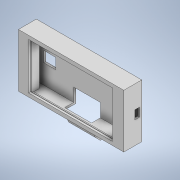
# Autodesk Inventor part: left
Saved by Autodesk Inventor 2020 (Build 240168000, 168)
## iProperties
Created: 2021-08-13
Part Number: left
Material: Generic
Document SubType Name: Modeling
Designer: khonsu
Density: 1 g/cm^3
Appearance: Default
Author: khonsu
Autodesk Inventor part; units mm, degrees
ref_plane "YZ Plane" through (0, 0, 0) normal (1, 0, 0) x (0, 1, 0)
ref_plane "XZ Plane" through (0, 0, 0) normal (0, 1, 0) x (-1, 0, 0)
ref_plane "XY Plane" through (0, 0, 0) normal (0, 0, 1) x (1, 0, 0)
sketch "Sketch1" plane through (0, 0, 0) normal (0, 0, 1) x (1, 0, 0)
  line L0 (0, 0) -> (74, 0)
  line L1 (74, 0) -> (74, -7.6)
  line L2 (74, -7.6) -> (0, -7.6)
  line L3 (0, -7.6) -> (0, 0)
  line L4 (0.9, 13.2) -> (73.1, 13.2)
  line L5 (73.1, 13.2) -> (73.1, 12)
  line L6 (73.1, 12) -> (0.9, 12)
  line L7 (0.9, 12) -> (0.9, 13.2)
  line L8 (-3, 16.2) -> (77, 16.2)
  line L9 (77, 16.2) -> (77, -10.6)
  line L10 (77, -10.6) -> (-3, -10.6)
  line L11 (-3, -10.6) -> (-3, 16.2)
  dimension "d0" = 74
  dimension "d1" = 7.6
  dimension "d2" = 1.2
  dimension "d3" = 12
  dimension "d4" = 72.2
  dimension "d5" = 0.9
  dimension "d6" = 3
  dimension "d7" = 3
  dimension "d8" = 3
  dimension "d9" = 3
  constraints: 24 end point, 6 parallel, 3 horizontal, 3 perpendicular
  measures "d0" distance of L0.start L0.end
  measures "d1" distance of L0.end L1.end
  measures "d2" distance of L4.end L5.end
  measures "d3" distance between parallel lines of L0 L6
  measures "d4" distance of L4.start L4.end
  measures "d5" distance between parallel lines of L3 L7
  measures "d6" distance between parallel lines of L8 L4
  measures "d7" distance between parallel lines of L2 L10
  measures "d8" distance between parallel lines of L3 L11
  measures "d9" distance between parallel lines of L9 L1
extrude "Extrusion1" add sketch "Sketch1" along normal blind 151.5
sketch "Sketch2" plane through (-3, 16.2, 0) normal (0, 1, 0) x (1, 0, 0)
  line L0 (77, -12.1) -> (3, -12.1)
  line L1 (3, -12.1) -> (3, -137.5)
  line L2 (3, -137.5) -> (77, -137.5)
  line L3 (77, -137.5) -> (77, -12.1)
  line L4 (80, 0) -> (80, -151.5) projected
  line L5 (0, 0) -> (0, -151.5) projected
  line L6 (80, 0) -> (0, 0) projected
  line L7 (80, -151.5) -> (0, -151.5) projected
  point P0 (3, 0)
  dimension "d12" = 3
  dimension "d14" = 12.1
  dimension "d15" = 14
  dimension "d23" = 3
  constraints: 8 end point, 2 parallel, 1 horizontal, 1 perpendicular
  measures "d12" distance between parallel lines of L4 L3
  measures "d14" distance between parallel lines of L6 L0
  measures "d15" distance between parallel lines of L7 L2
  measures "d23" distance between parallel lines of L5 L1
extrude "Extrusion2" cut sketch "Sketch2" against normal up to surface (23.8 mm away) contours L3 L2 L1 L0
sketch "Sketch3" plane through (-3, 16.2, 0) normal (0, 1, 0) x (1, 0, 0)
  line L0 (80, 0) -> (80, -151.5) projected
  line L1 (0, 0) -> (0, -151.5) projected
  line L2 (80, -0.75) -> (0, -0.75)
  line L3 (0, -0.75) -> (0, -150.75)
  line L4 (0, -150.75) -> (80, -150.75)
  line L5 (80, -150.75) -> (80, -0.75)
  line L6 (80, -151.5) -> (0, -151.5) projected
  line L7 (80, 0) -> (0, 0) projected
  line L8 (80, 0) -> (0, 0)
  line L9 (0, 0) -> (0, -151.5)
  line L10 (0, -151.5) -> (80, -151.5)
  line L11 (80, -151.5) -> (80, 0)
  point P0 (3, 0)
  point P1 (0, -0.75)
  dimension "d18" = 150
  dimension "d19" = 151.5
  dimension "d20" = 0.75
  constraints: 16 end point, 4 parallel, 2 horizontal, 2 perpendicular, 2 point on line
  measures "d18" distance between parallel lines of L4 L2
  measures "d19" distance of L0.start L0.end
  measures "d20" distance between parallel lines of L6 L4
extrude "Extrusion3" add sketch "Sketch3" against normal up to surface (4.2 mm away) contours L0 L2 L1 L7 | L0 L6 L1 L4
sketch "Sketch4" plane through (0, 0, 0) normal (0, 0, -1) x (-1, 0, 0)
  line L0 (-77, -10.6) -> (-77, 16.2) projected
  line L1 (3, 16.2) -> (3, -10.6) projected
  line L2 (-77, -10.6) -> (3, -10.6)
  line L3 (3, -10.6) -> (3, 16.2)
  line L4 (3, 16.2) -> (-77, 16.2)
  line L5 (-77, 16.2) -> (-77, -10.6)
  point P0 (0, 0)
  constraints: 8 end point, 2 parallel, 1 horizontal, 1 perpendicular
extrude "Extrusion4" add sketch "Sketch4" along normal blind 3
sketch "Sketch5" plane through (0, 0, 151.5) normal (0, 0, 1) x (1, 0, 0)
  line L0 (-3, 16.2) -> (77, 16.2) projected
  line L1 (77, -10.6) -> (-3, -10.6) projected
  line L2 (77, 16.2) -> (-3, 16.2)
  line L3 (-3, 16.2) -> (-3, -10.6)
  line L4 (-3, -10.6) -> (77, -10.6)
  line L5 (77, -10.6) -> (77, 16.2)
  line L6 (43.5, -0.4) -> (30.5, -0.4)
  line L7 (30.5, -0.4) -> (30.5, -7.2)
  line L8 (30.5, -7.2) -> (43.5, -7.2)
  line L9 (43.5, -7.2) -> (43.5, -0.4)
  line L10 (74, -7.6) -> (0, -7.6) projected
  line L11 (74, 0) -> (74, -7.6) projected
  point P0 (0, 0)
  dimension "d26" = 6.8
  dimension "d27" = 13
  dimension "d28" = 0.4
  dimension "d29" = 30.5
  constraints: 16 end point, 4 parallel, 2 horizontal, 2 perpendicular
  measures "d26" distance of L8.end L6.start
  measures "d27" distance of L7.end L8.end
  measures "d28" distance between parallel lines of L10 L8
  measures "d29" distance between parallel lines of L11 L9
extrude "Extrusion5" add sketch "Sketch5" along normal blind 3
sketch "Sketch6" plane through (-3, -10.6, -3) normal (0, -1, 0) x (1, 0, 0)
  line L0 (48, 14.3) -> (32, 14.3)
  line L1 (32, 14.3) -> (32, 32)
  line L2 (32, 32) -> (48, 32)
  line L3 (48, 32) -> (48, 14.3)
  line L4 (77, 3) -> (3, 3) projected
  line L5 (80, 157.5) -> (80, 0) projected
  dimension "d32" = 11.3
  dimension "d33" = 16
  dimension "d34" = 17.7
  dimension "d35" = 32
  constraints: 8 end point, 2 parallel, 1 horizontal, 1 perpendicular
  measures "d32" distance between parallel lines of L4 L0
  measures "d33" distance of L0.start L0.end
  measures "d34" distance of L2.end L0.start
  measures "d35" distance between parallel lines of L5 L3
extrude "Extrusion6" cut sketch "Sketch6" against normal up to surface (3 mm away)
sketch "Sketch7" plane through (-3, 16.2, -3) normal (0, 1, 0) x (1, 0, 0)
  line L0 (3, -15.1) -> (77, -15.1) projected
  line L1 (77, -140.5) -> (3, -140.5) projected
  line L2 (74.6, -15.1) -> (5.4, -15.1)
  line L3 (5.4, -15.1) -> (5.4, -140.5)
  line L4 (5.4, -140.5) -> (74.6, -140.5)
  line L5 (74.6, -140.5) -> (74.6, -15.1)
  line L6 (77, -15.1) -> (77, -140.5) projected
  line L7 (3, -140.5) -> (3, -15.1) projected
  line L8 (77, -3) -> (77, -15.1) projected
  line L9 (77, -15.1) -> (3, -15.1)
  line L10 (3, -15.1) -> (3, -140.5)
  line L11 (3, -140.5) -> (77, -140.5)
  line L12 (77, -140.5) -> (77, -15.1)
  point P0 (3, -3)
  point P1 (5.4, -15.1)
  dimension "d38" = 2.4
  dimension "d39" = 2.4
  constraints: 16 end point, 4 parallel, 2 horizontal, 2 perpendicular, 2 point on line
  measures "d38" distance between parallel lines of L6 L5
  measures "d39" distance between parallel lines of L7 L3
extrude "Extrusion7" add sketch "Sketch7" against normal up to surface (3 mm away) contours L0 L3 L1 L7 | L0 L6 L1 L5
sketch "Sketch8" plane through (0, 0, -3) normal (0, 0, -1) x (-1, 0, 0)
  line L0 (-74, -7.6) -> (0, -7.6) projected
  line L1 (-18.5, -7.6) -> (-28.5, -7.6)
  line L2 (-31, -5.1) -> (-31, -5.1)
  line L3 (-28.5, -2.6) -> (-18.5, -2.6)
  line L4 (-16, -5.1) -> (-16, -5.1)
  line L5 (0, -7.6) -> (0, 0) projected
  line L6 (0, 0) -> (-74, 0) projected
  arc A0 (-31, -5.1) -> (-28.5, -7.6) centre (-28.5, -5.1) ccw
  arc A1 (-28.5, -2.6) -> (-31, -5.1) centre (-28.5, -5.1) ccw
  arc A2 (-18.5, -7.6) -> (-16, -5.1) centre (-18.5, -5.1) ccw
  arc A3 (-16, -5.1) -> (-18.5, -2.6) centre (-18.5, -5.1) ccw
  point P0 (-16, -7.6)
  point P1 (-31, -2.6)
  point P2 (-31, -7.6)
  point P3 (-16, -2.6)
  dimension "d42" = 15
  dimension "d43" = 16
  dimension "d44" = 2.6
  dimension "d45" = 5
  dimension "d46" = 2.5
  constraints: 9 point on line, 8 end point, 8 point on circle, 8 tangent, 4 centre point, 3 equal radius, 2 parallel, 1 horizontal, 1 perpendicular
  measures "d42" distance of point (-31, -2.6) point (-16, -2.6)
  measures "d43" distance between parallel lines of L5 L4
  measures "d44" distance between parallel lines of L6 L3
  measures "d45" distance of point (-31, -7.6) point (-31, -2.6)
  measures "d46" radius of A0
extrude "Extrusion8" cut sketch "Sketch8" against normal up to surface (3 mm away)
sketch "Sketch9" plane through (0, 0, 12.1) normal (0, 0, 1) x (1, 0, 0)
  line L0 (0.9, 12) -> (0.9, 13.2) projected
  line L1 (0.9, 12) -> (0, 12)
  line L2 (0, 13.2) -> (0, 0) projected
  line L3 (0, 12) -> (1.9, 12)
  line L4 (1.9, 12) -> (1.9, 10.5)
  line L5 (1.9, 10.5) -> (0, 10.5)
  line L6 (0, 10.5) -> (0, 12)
  line L7 (0.9, 13.2) -> (0, 13.2)
  line L8 (0, 13.2) -> (0, 12)
  line L9 (0, 12) -> (0.9, 12)
  line L10 (0.9, 12) -> (0.9, 13.2)
  line L11 (73.1, 12) -> (73.1, 13.2) projected
  line L12 (73.1, 12) -> (74, 12)
  line L13 (74, 13.2) -> (74, 0) projected
  line L14 (74, 12) -> (72.1, 12)
  line L15 (72.1, 12) -> (72.1, 10.5)
  line L16 (72.1, 10.5) -> (74, 10.5)
  line L17 (74, 10.5) -> (74, 12)
  line L18 (74, 13.2) -> (73.1, 13.2) projected
  line L19 (73.1, 12) -> (74, 12)
  line L20 (74, 12) -> (74, 13.2)
  line L21 (74, 13.2) -> (73.1, 13.2)
  line L22 (73.1, 13.2) -> (73.1, 12)
  point P0 (0, 10.5)
  point P1 (73.1, 12)
  dimension "d49" = 1
  dimension "d50" = 1.5
  dimension "d52" = 1.5
  dimension "d53" = 1
  constraints: 36 end point, 8 parallel, 6 horizontal, 4 perpendicular, 2 point on line
  measures "d49" distance between parallel lines of L0 L4
  measures "d50" distance of L3.end L4.end
  measures "d52" distance of L15.end L14.end
  measures "d53" distance between parallel lines of L11 L15
extrude "Extrusion9" add sketch "Sketch9" along normal up to surface (125.4 mm away)
sketch "Sketch10" plane through (-3, -10.6, -3) normal (0, -1, 0) x (1, 0, 0)
  line L0 (20, 98.75) -> (-20, 98.75)
  line L1 (-20, 98.75) -> (-20, 58.75)
  line L2 (-20, 58.75) -> (20, 58.75)
  line L3 (20, 58.75) -> (20, 98.75)
  line L4 (80, 0) -> (0, 0) projected
  line L5 (0, 0) -> (0, 157.5) projected
  point P0 (3, 3)
  dimension "d56" = 40
  dimension "d57" = 40
  dimension "d58" = 58.75
  dimension "d59" = 20
  constraints: 8 end point, 2 parallel, 1 horizontal, 1 perpendicular
  measures "d56" distance of L2.end L1.end
  measures "d57" distance of L1.end L0.end
  measures "d58" distance between parallel lines of L4 L2
  measures "d59" distance between parallel lines of L5 L3
extrude "Extrusion10" cut sketch "Sketch10" against normal blind 13.4
chamfer "Chamfer1" distance 3 angle 45 1 edges at (17, -7.6, 75.75)
sketch "Sketch12" plane through (-3, -10.6, 55.75) normal (0, 0, 1) x (1, 0, 0)
  line L0 (-17.0576, 7.8863) -> (11.2267, -20.3979)
  line L1 (11.2267, -20.3979) -> (4.1557, -27.469)
  line L2 (4.1557, -27.469) -> (-24.1286, 0.8153)
  line L3 (-24.1286, 0.8153) -> (-17.0576, 7.8863)
  line L4 (80, 0) -> (0, 0) projected
  line L5 (0, 13.4) -> (3, 16.4) projected
  line L6 (3, 16.4) -> (-17.0576, 7.8863)
  line L7 (23, 3) -> (20, 0) projected
  line L8 (23, 3) -> (11.2267, -20.3979)
  line L9 (23, 3) -> (3, 16.4)
  point P0 (3, 10.6)
  point P1 (21.4905, 0)
  dimension "d65" = 90
  dimension "d66" = 90
  dimension "d67" = 45
  dimension "d68" = 10
  dimension "d69" = 40
  constraints: 14 end point, 3 perpendicular
  measures "d65" angle of L1 L0
  measures "d66" angle of L2 L3
  measures "d67" angle of L4 L0
  measures "d68" distance between parallel lines of L2 L0
  measures "d69" distance between parallel lines of L3 L1
extrude "Extrusion11" cut sketch "Sketch12" along normal up to surface (40 mm away) contours L6 L9 L7 L4 L8 L0 | L4 L7 L8
sketch "Sketch13" plane through (-3, -10.6, 55.75) normal (0, 0, 1) x (1, 0, 0)
  line L0 (-17.0576, 7.8863) -> (11.2267, -20.3979)
  line L1 (11.2267, -20.3979) -> (4.1557, -27.469)
  line L2 (4.1557, -27.469) -> (-24.1286, 0.8153)
  line L3 (-24.1286, 0.8153) -> (-17.0576, 7.8863)
  line L4 (3, 16.4) -> (-17.0576, 7.8863)
  line L5 (23, 3) -> (11.2267, -20.3979)
  line L6 (23, 3) -> (3, 16.4) construction
  line L7 (-18.1567, 11.0298) -> (-26.2499, 2.9366)
  line L8 (-28.3713, 0.8153) -> (4.1557, -31.7116) construction
  line L9 (6.277, -29.5903) -> (18.682, -17.1853)
  line L10 (-24.1286, 0.8153) -> (-26.2499, 2.9366)
  line L11 (-26.2499, 2.9366) -> (6.277, -29.5903)
  line L12 (-1.8502, 17.6004) -> (-8.6324, 14.7216)
  line L13 (-1.8502, 17.6004) -> (-22.9463, 8.6459)
  line L14 (-9.9896, 14.1455) -> (3.638, 19.9299)
  line L15 (0, 0) -> (0, 26.8) projected
  line L16 (0, 15.1266) -> (0, 18.3857)
  line L17 (0, 0) -> (0, 15.1266) projected
  line L18 (23.2213, -3.2345) -> (18.7952, -12.0308)
  line L19 (23.2213, -3.2345) -> (9.1734, -31.1531)
  line L20 (17.9281, -13.7542) -> (27.2379, 4.7479)
  line L21 (80, 0) -> (0, 0) projected
  line L22 (24.8488, 0) -> (21.4905, 0)
  point P0 (3, 10.6)
  point P1 (4, 11.6)
  point P2 (0, 18.3857)
  point P3 (-8.6324, 14.7216)
  point P4 (-18.7665, 10.42)
  point P5 (13.6895, -22.1778)
  point P6 (23.2213, -3.2345)
  dimension "d72" = 90
  dimension "d73" = 90
  dimension "d74" = 10
  dimension "d75" = 40
  dimension "d76" = 3
  dimension "d77" = 3
  dimension "d78" = 3
  dimension "d79" = 3
  dimension "d80" = 3
  constraints: 40 end point, 10 point on line, 5 collinear, 5 perpendicular, 3 parallel
  measures "d72" angle of L1 L0
  measures "d73" angle of L2 L3
  measures "d74" distance between parallel lines of L2 L0
  measures "d75" distance between parallel lines of L3 L1
  measures "d76" distance between parallel lines of L3 L7
  measures "d77" distance between parallel lines of L2 L8
  measures "d78" distance between parallel lines of L1 L9
  measures "d79" distance between parallel lines of L4 L12
  measures "d80" distance between parallel lines of L5 L18
extrude "Extrusion12" add sketch "Sketch13" along normal up to surface (40 mm away) contours L3 L10 L7 L13 L12 L14 L15 L4 | L5 L21 L20 L18 L19 L9 L11 L1
body "Solid1"
